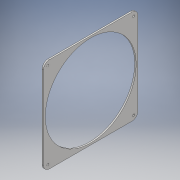
# Autodesk Inventor part: TrayPanelD_180mm
Saved by Autodesk Inventor 2017 (Build 210142000, 142)
## iProperties
Created: 2019-06-22
Part Number: TrayPanelD_180mm
Material: Generic
Document SubType Name: Modeling
Designer: DDeGo
Density: 1 g/cm^3
Appearance: Default
Author: DDeGo
Autodesk Inventor part; units mm, degrees
ref_plane "YZ Plane" through (0, 0, 0) normal (1, 0, 0) x (0, 1, 0)
ref_plane "XZ Plane" through (0, 0, 0) normal (0, 1, 0) x (-1, 0, 0)
ref_plane "XY Plane" through (0, 0, 0) normal (0, 0, 1) x (1, 0, 0)
sketch "Sketch1" plane through (0, 0, 0) normal (1, 0, 0) x (0, 1, 0)
  circle A0 centre (5.5, -2.5) radius 2
  circle A1 centre (88, 80) radius 87.5
  circle A2 centre (170.5, -2.5) radius 2
  circle A3 centre (5.5, 162.5) radius 2
  circle A4 centre (170.5, 162.5) radius 2
  line L0 (167.5, 171) -> (8.5, 171)
  arc A5 (8.5, 171) -> (-3, 159.5) centre (8.5, 159.5) ccw
  line L1 (-3, 159.5) -> (-3, 0.5)
  arc A6 (-3, 0.5) -> (8.5, -11) centre (8.5, 0.5) ccw
  line L2 (8.5, -11) -> (167.5, -11)
  arc A7 (167.5, -11) -> (179, 0.5) centre (167.5, 0.5) ccw
  line L3 (179, 0.5) -> (179, 159.5)
  arc A8 (179, 159.5) -> (167.5, 171) centre (167.5, 159.5) ccw
  point P0 (0, 0)
  point P1 (183, -15)
  constraints: 9 centre point, 8 end point, 8 point on circle
extrude "Extrusion1" add sketch "Sketch1" along normal blind 2.75
body "Solid1"
